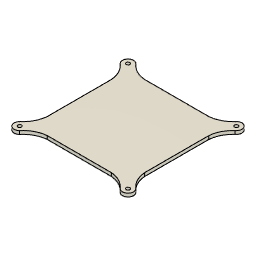
Rockin-Base (Autodesk Fusion 360 design; units mm, degrees)
Autodesk Fusion 360 part; units mm, degrees
sketch "RockinBase" plane through (-30.9845, 0, -2.9179) normal (0, 1, 0) x (-1, 0, 0)
  line L0 (109, -95) -> (109, 95)
  arc A0 (109, 95) -> (106, 98) centre (106, 95) ccw
  line L1 (106, 98) -> (-106, 98)
  arc A1 (-106, 98) -> (-109, 95) centre (-106, 95) ccw
  line L2 (-109, 95) -> (-109, -95)
  arc A2 (-109, -95) -> (-106, -98) centre (-106, -95) ccw
  line L3 (-106, -98) -> (106, -98)
  arc A3 (106, -98) -> (109, -95) centre (106, -95) ccw
  circle A4 centre (95.5, -84.5) radius 5
  circle A5 centre (95.5, 84.5) radius 5
  line L4 (-72.9845, 44) -> (11.0155, 44)
  line L5 (11.0155, -44) -> (-72.9845, -44)
  line L6 (13.0155, 42) -> (13.0155, -42)
  line L7 (-74.9845, -42) -> (-74.9845, 42)
  circle A6 centre (-79.9845, 49) radius 2.05
  circle A7 centre (-79.9845, -49) radius 2.05
  circle A8 centre (18.0155, -49) radius 2.05
  circle A9 centre (18.0155, 49) radius 2.05
  arc A10 (13.0155, 42) -> (11.0155, 44) centre (11.0155, 42) ccw
  arc A11 (11.0155, -44) -> (13.0155, -42) centre (11.0155, -42) ccw
  arc A12 (-72.9845, 44) -> (-74.9845, 42) centre (-72.9845, 42) ccw
  arc A13 (-74.9845, -42) -> (-72.9845, -44) centre (-72.9845, -42) ccw
  circle A14 centre (18.0155, -49) radius 5.05
  circle A15 centre (-79.9845, -49) radius 5.05
  circle A16 centre (-79.9845, 49) radius 5.05
  circle A17 centre (18.0155, 49) radius 5.05
  line L8 (25, -49) -> (10, -49) construction
  line L9 (18.0155, -54.05) -> (18.0155, -42) construction
  line L10 (21.6242, -45.4673) -> (14.4828, -52.6087) construction
  line L11 (21.5674, -52.5898) -> (14.4257, -45.4481) construction
  arc A18 (13.0155, -29) -> (21.6242, -45.4673) centre (36.614, -27.1472) ccw
  line L12 (13.0155, -29) -> (21.6242, -29) construction
  line L13 (21.6242, -29) -> (21.6242, -45.4673) construction
  line L14 (-1.9845, -44) -> (-1.9845, -52.6087) construction
  line L15 (-1.9845, -52.6087) -> (14.4828, -52.6087) construction
  line L16 (21.9548, -39) -> (13.0155, -39) construction
  line L17 (8.0155, -44) -> (8.0155, -52.6087) construction
  line L18 (16.1242, -39) -> (16.1242, -29) construction
  line L19 (8.0094, -47.1087) -> (-1.9845, -47.1087) construction
  arc A19 (14.4828, -52.6087) -> (-1.9845, -44) centre (-3.855, -67.6323) ccw
  arc A20 (21.6242, 45.4673) -> (13.0155, 29) centre (36.614, 27.1472) ccw
  arc A21 (-1.9845, 44) -> (14.4828, 52.6087) centre (-3.855, 67.6323) ccw
  circle A22 centre (-95.5, -84.5) radius 5
  circle A23 centre (-95.5, 84.5) radius 5
  circle A24 centre (18.0155, 49) radius 2.05
  circle A25 centre (-79.9845, 49) radius 2.05
  circle A26 centre (18.0155, -49) radius 2.05
  circle A27 centre (-79.9845, -49) radius 2.05
  line L20 (-72.9845, 44) -> (11.0155, 44)
  arc A28 (13.0155, 42) -> (11.0155, 44) centre (11.0155, 42) ccw
  line L21 (13.0155, 42) -> (13.0155, -42)
  arc A29 (11.0155, -44) -> (13.0155, -42) centre (11.0155, -42) ccw
  line L22 (11.0155, -44) -> (-72.9845, -44)
  arc A30 (-74.9845, -42) -> (-72.9845, -44) centre (-72.9845, -42) ccw
  line L23 (-74.9845, -42) -> (-74.9845, 42)
  arc A31 (-72.9845, 44) -> (-74.9845, 42) centre (-72.9845, 42) ccw
  line L24 (49.9363, -38.9018) -> (49.9363, -43.5825)
  line L25 (49.9363, -43.5825) -> (31.9363, -43.5825)
  line L26 (31.9363, -43.5825) -> (31.9363, -40.2693)
  spline S0 degree 3 poles (31.9363, -40.2693) (31.9322, -39.3416) (31.9257, -37.84) (32.1184, -36.3519) (32.192, -35.7832) knots 0 0 0 0 0.277884 0.449757 0.449757 0.449757 0.449757
  spline S1 degree 3 poles (32.192, -35.7832) (32.3135, -35.4081) (32.5613, -34.6434) (33.1821, -34.1316) (33.4984, -33.8709) knots 0 0 0 0 0.115749 0.235933 0.235933 0.235933 0.235933
  spline S2 degree 3 poles (33.4984, -33.8709) (33.9456, -33.6565) (34.9997, -33.1511) (36.1742, -33.1387) (36.8504, -33.1316) knots 0 0 0 0 0.14718 0.346909 0.346909 0.346909 0.346909
  spline S3 degree 3 poles (36.8504, -33.1316) (37.4464, -33.1268) (38.4271, -33.1191) (39.323, -33.5034) (39.6744, -33.6541) knots 0 0 0 0 0.176149 0.289849 0.289849 0.289849 0.289849
  spline S4 degree 3 poles (39.6744, -33.6541) (39.8929, -33.9007) (40.4082, -34.4822) (40.4928, -35.2619) (40.5416, -35.7109) knots 0 0 0 0 0.096727 0.228082 0.228082 0.228082 0.228082
  spline S5 degree 3 poles (40.5416, -35.7109) (40.6442, -35.307) (40.82, -34.615) (41.275, -34.07) (41.4644, -33.8431) knots 0 0 0 0 0.122975 0.210643 0.210643 0.210643 0.210643
  spline S6 degree 3 poles (41.4644, -33.8431) (41.6426, -33.7017) (41.9651, -33.4458) (42.3527, -33.3094) (42.5262, -33.2483) knots 0 0 0 0 0.067663 0.122452 0.122452 0.122452 0.122452
  spline S7 degree 3 poles (42.5262, -33.2483) (42.8284, -33.215) (43.7127, -33.1175) (44.603, -33.126) (45.1889, -33.1316) knots 0 0 0 0 0.091172 0.266721 0.266721 0.266721 0.266721
  line L27 (45.1889, -33.1316) -> (49.9363, -33.1316)
  line L28 (49.9363, -33.1316) -> (49.9363, -37.4787)
  line L29 (49.9363, -37.4787) -> (43.9548, -37.4787)
  spline S8 degree 3 poles (43.9548, -37.4787) (43.5604, -37.4703) (42.9494, -37.4573) (42.3701, -37.6414) (42.1648, -37.7066) knots 0 0 0 0 0.117155 0.181452 0.181452 0.181452 0.181452
  spline S9 degree 3 poles (42.1648, -37.7066) (42.0656, -37.8397) (41.806, -38.1877) (41.8147, -38.6291) (41.8202, -38.9018) knots 0 0 0 0 0.048702 0.127417 0.127417 0.127417 0.127417
  line L30 (41.8202, -38.9018) -> (49.9363, -38.9018)
  spline S10 degree 3 poles (35.6608, -11.9518) (35.9149, -11.5755) (36.3988, -10.8588) (37.1724, -10.4767) (37.5397, -10.2952) knots 0 0 0 0 0.133571 0.254362 0.254362 0.254362 0.254362
  spline S11 degree 3 poles (37.5397, -10.2952) (37.9942, -10.1758) (39.0458, -9.8995) (40.1346, -9.8895) (40.7528, -9.8839) knots 0 0 0 0 0.140459 0.325027 0.325027 0.325027 0.325027
  line L31 (40.7528, -9.8839) -> (40.7528, -14.1198)
  line L32 (40.7528, -14.1198) -> (39.0518, -14.1198)
  spline S12 degree 3 poles (39.0518, -14.1198) (38.8011, -14.1181) (38.3918, -14.1152) (37.998, -14.2227) (37.8455, -14.2644) knots 0 0 0 0 0.074717 0.121977 0.121977 0.121977 0.121977
  spline S13 degree 3 poles (37.8455, -14.2644) (37.7531, -14.3249) (37.5615, -14.4504) (37.5398, -14.6795) (37.5286, -14.798) knots 0 0 0 0 0.03143 0.06517 0.06517 0.06517 0.06517
  spline S14 degree 3 poles (37.5286, -14.798) (37.5364, -14.9151) (37.5509, -15.1331) (37.7256, -15.2612) (37.8066, -15.3206) knots 0 0 0 0 0.033254 0.06196 0.06196 0.06196 0.06196
  spline S15 degree 3 poles (37.8066, -15.3206) (37.956, -15.3589) (38.3632, -15.4632) (38.7849, -15.4576) (39.0518, -15.454) knots 0 0 0 0 0.046126 0.12569 0.12569 0.12569 0.12569
  line L33 (39.0518, -15.454) -> (46.0116, -15.454)
  spline S16 degree 3 poles (46.0116, -15.454) (46.2446, -15.4518) (46.6509, -15.4479) (47.0327, -15.3119) (47.1957, -15.2539) knots 0 0 0 0 0.069251 0.12082 0.12082 0.12082 0.12082
  spline S17 degree 3 poles (47.1957, -15.2539) (47.3108, -15.1821) (47.532, -15.0441) (47.5714, -14.7877) (47.5904, -14.6646) knots 0 0 0 0 0.038577 0.07416 0.07416 0.07416 0.07416
  spline S18 degree 3 poles (47.5904, -14.6646) (47.574, -14.5252) (47.5414, -14.2493) (47.299, -14.1143) (47.179, -14.0476) knots 0 0 0 0 0.039578 0.078352 0.078352 0.078352 0.078352
  spline S19 degree 3 poles (47.179, -14.0476) (46.9815, -14.0011) (46.4708, -13.881) (45.945, -13.8843) (45.6225, -13.8864) knots 0 0 0 0 0.060698 0.156952 0.156952 0.156952 0.156952
  line L34 (45.6225, -13.8864) -> (43.8659, -13.8864)
  line L35 (43.8659, -13.8864) -> (43.8659, -9.8839)
  spline S20 degree 3 poles (43.8659, -9.8839) (44.3819, -9.8878) (45.2677, -9.8945) (46.1495, -9.9772) (46.5175, -10.0117) knots 0 0 0 0 0.154724 0.265578 0.265578 0.265578 0.265578
  spline S21 degree 3 poles (46.5175, -10.0117) (46.8221, -10.0776) (47.4698, -10.2177) (48.032, -10.57) (48.3297, -10.7566) knots 0 0 0 0 0.092782 0.197263 0.197263 0.197263 0.197263
  spline S22 degree 3 poles (48.3297, -10.7566) (48.6201, -10.9818) (49.2003, -11.4318) (49.5539, -12.0752) (49.7306, -12.3965) knots 0 0 0 0 0.108972 0.217725 0.217725 0.217725 0.217725
  spline S23 degree 3 poles (49.7306, -12.3965) (49.8682, -12.7698) (50.1655, -13.5761) (50.19, -14.4361) (50.2031, -14.8981) knots 0 0 0 0 0.118546 0.256084 0.256084 0.256084 0.256084
  spline S24 degree 3 poles (50.2031, -14.8981) (50.1888, -15.4752) (50.1629, -16.5234) (49.7419, -17.4808) (49.5527, -17.9111) knots 0 0 0 0 0.171157 0.310864 0.310864 0.310864 0.310864
  spline S25 degree 3 poles (49.5527, -17.9111) (49.3153, -18.2541) (48.8433, -18.9362) (48.0992, -19.3023) (47.7294, -19.4843) knots 0 0 0 0 0.122923 0.244404 0.244404 0.244404 0.244404
  spline S26 degree 3 poles (47.7294, -19.4843) (47.2592, -19.6182) (46.1727, -19.9278) (45.0413, -19.9392) (44.3995, -19.9456) knots 0 0 0 0 0.146052 0.33749 0.33749 0.33749 0.33749
  line L36 (44.3995, -19.9456) -> (40.2081, -19.9456)
  spline S27 degree 3 poles (40.2081, -19.9456) (39.6546, -19.9419) (38.692, -19.9352) (37.7664, -19.6773) (37.373, -19.5676) knots 0 0 0 0 0.165095 0.287118 0.287118 0.287118 0.287118
  spline S28 degree 3 poles (37.373, -19.5676) (37.0535, -19.3898) (36.3506, -18.9987) (35.9079, -18.3237) (35.6664, -17.9555) knots 0 0 0 0 0.108122 0.237874 0.237874 0.237874 0.237874
  spline S29 degree 3 poles (35.6664, -17.9555) (35.4476, -17.5077) (34.9856, -16.5617) (34.9399, -15.5084) (34.9159, -14.9537) knots 0 0 0 0 0.147881 0.312389 0.312389 0.312389 0.312389
  spline S30 degree 3 poles (34.9159, -14.9537) (34.9402, -14.4011) (34.9865, -13.3489) (35.4437, -12.4016) (35.6608, -11.9518) knots 0 0 0 0 0.163939 0.312177 0.312177 0.312177 0.312177
  line L37 (35.5385, 37.6788) -> (33.2148, 37.6788)
  line L38 (33.2148, 37.6788) -> (33.2148, 42.1816)
  line L39 (33.2148, 42.1816) -> (35.5385, 42.1816)
  line L40 (35.5385, 42.1816) -> (35.5385, 43.3935)
  line L41 (35.5385, 43.3935) -> (37.8733, 43.3935)
  line L42 (37.8733, 43.3935) -> (37.8733, 42.1816)
  line L43 (37.8733, 42.1816) -> (45.767, 42.1816)
  spline S31 degree 3 poles (45.767, 42.1816) (46.1483, 42.169) (46.6983, 42.1509) (47.2278, 42.2893) (47.3903, 42.3317) knots 0 0 0 0 0.113465 0.163663 0.163663 0.163663 0.163663
  spline S32 degree 3 poles (47.3903, 42.3317) (47.4376, 42.4599) (47.5853, 42.8601) (47.5685, 43.2902) (47.557, 43.5825) knots 0 0 0 0 0.040741 0.127145 0.127145 0.127145 0.127145
  line L44 (47.557, 43.5825) -> (49.9363, 43.5825)
  line L45 (49.9363, 43.5825) -> (49.9363, 41.7702)
  spline S33 degree 3 poles (49.9363, 41.7702) (49.9367, 41.3313) (49.9375, 40.5983) (49.8454, 39.8715) (49.8084, 39.58) knots 0 0 0 0 0.131509 0.219587 0.219587 0.219587 0.219587
  spline S34 degree 3 poles (49.8084, 39.58) (49.7515, 39.3674) (49.6372, 38.9402) (49.359, 38.5964) (49.2192, 38.4237) knots 0 0 0 0 0.06522 0.131072 0.131072 0.131072 0.131072
  spline S35 degree 3 poles (49.2192, 38.4237) (49.063, 38.2734) (48.76, 37.9817) (48.3579, 37.8601) (48.163, 37.8011) knots 0 0 0 0 0.063989 0.124175 0.124175 0.124175 0.124175
  spline S36 degree 3 poles (48.163, 37.8011) (47.8311, 37.7661) (46.9021, 37.6681) (45.9675, 37.6746) (45.3668, 37.6788) knots 0 0 0 0 0.100066 0.280064 0.280064 0.280064 0.280064
  line L46 (45.3668, 37.6788) -> (37.8733, 37.6788)
  line L47 (37.8733, 37.6788) -> (37.8733, 36.7116)
  line L48 (37.8733, 36.7116) -> (35.5385, 36.7116)
  line L49 (35.5385, 36.7116) -> (35.5385, 37.6788)
  line L50 (49.9363, 13.9753) -> (31.9363, 13.9753)
  line L51 (31.9363, 13.9753) -> (31.9363, 18.467)
  line L52 (31.9363, 18.467) -> (36.1972, 18.467)
  spline S37 degree 3 poles (36.1972, 18.467) (35.9973, 18.6537) (35.6098, 19.0158) (35.3562, 19.4813) (35.2335, 19.7066) knots 0 0 0 0 0.081471 0.157931 0.157931 0.157931 0.157931
  spline S38 degree 3 poles (35.2335, 19.7066) (35.1408, 19.9414) (34.9527, 20.4184) (34.9283, 20.9307) (34.9159, 21.1909) knots 0 0 0 0 0.075167 0.152706 0.152706 0.152706 0.152706
  spline S39 degree 3 poles (34.9159, 21.1909) (34.9249, 21.4809) (34.942, 22.0293) (35.1207, 22.5476) (35.205, 22.7918) knots 0 0 0 0 0.086467 0.163515 0.163515 0.163515 0.163515
  spline S40 degree 3 poles (35.205, 22.7918) (35.3072, 23.0018) (35.5037, 23.4053) (35.8503, 23.6895) (36.0166, 23.8258) knots 0 0 0 0 0.069125 0.132834 0.132834 0.132834 0.132834
  spline S41 degree 3 poles (36.0166, 23.8258) (36.1844, 23.9317) (36.5017, 24.132) (36.8672, 24.2148) (37.0394, 24.2539) knots 0 0 0 0 0.059029 0.111602 0.111602 0.111602 0.111602
  spline S42 degree 3 poles (37.0394, 24.2539) (37.3006, 24.2746) (38.0108, 24.331) (38.7235, 24.328) (39.1741, 24.3261) knots 0 0 0 0 0.078569 0.213664 0.213664 0.213664 0.213664
  line L53 (39.1741, 24.3261) -> (45.8226, 24.3261)
  spline S43 degree 3 poles (45.8226, 24.3261) (46.2964, 24.3248) (47.1094, 24.3226) (47.9076, 24.1721) (48.2408, 24.1093) knots 0 0 0 0 0.141719 0.24323 0.24323 0.24323 0.24323
  spline S44 degree 3 poles (48.2408, 24.1093) (48.5013, 24.0066) (49.0498, 23.7903) (49.4233, 23.3324) (49.6194, 23.092) knots 0 0 0 0 0.082602 0.173904 0.173904 0.173904 0.173904
  spline S45 degree 3 poles (49.6194, 23.092) (49.7896, 22.8078) (50.14, 22.2226) (50.1817, 21.5412) (50.2031, 21.1909) knots 0 0 0 0 0.097889 0.201485 0.201485 0.201485 0.201485
  spline S46 degree 3 poles (50.2031, 21.1909) (50.1892, 20.933) (50.1615, 20.4214) (49.9585, 19.9511) (49.8578, 19.7177) knots 0 0 0 0 0.076784 0.152376 0.152376 0.152376 0.152376
  spline S47 degree 3 poles (49.8578, 19.7177) (49.724, 19.4912) (49.4454, 19.0195) (49.035, 18.6559) (48.8217, 18.467) knots 0 0 0 0 0.078411 0.163305 0.163305 0.163305 0.163305
  line L54 (48.8217, 18.467) -> (49.9363, 18.1779)
  line L55 (49.9363, 18.1779) -> (49.9363, 13.9753)
  spline S48 degree 3 poles (36.5391, 34.9438) (36.7763, 35.1231) (37.2322, 35.4677) (37.7706, 35.6584) (38.0289, 35.7498) knots 0 0 0 0 0.088578 0.170285 0.170285 0.170285 0.170285
  spline S49 degree 3 poles (38.0289, 35.7498) (38.3505, 35.8127) (39.1206, 35.9631) (39.9061, 35.9653) (40.3637, 35.9666) knots 0 0 0 0 0.098084 0.234942 0.234942 0.234942 0.234942
  line L56 (40.3637, 35.9666) -> (43.977, 35.9666)
  spline S50 degree 3 poles (43.977, 35.9666) (44.5532, 35.9662) (45.5311, 35.9654) (46.4982, 35.8244) (46.8955, 35.7665) knots 0 0 0 0 0.17254 0.292859 0.292859 0.292859 0.292859
  spline S51 degree 3 poles (46.8955, 35.7665) (47.2029, 35.6784) (47.8324, 35.4978) (48.3599, 35.1093) (48.6299, 34.9104) knots 0 0 0 0 0.095113 0.194798 0.194798 0.194798 0.194798
  spline S52 degree 3 poles (48.6299, 34.9104) (48.8819, 34.6739) (49.3932, 34.1938) (49.6761, 33.5517) (49.8195, 33.2261) knots 0 0 0 0 0.102553 0.208104 0.208104 0.208104 0.208104
  spline S53 degree 3 poles (49.8195, 33.2261) (49.9313, 32.8604) (50.1667, 32.0909) (50.1906, 31.286) (50.2031, 30.8635) knots 0 0 0 0 0.114169 0.240306 0.240306 0.240306 0.240306
  spline S54 degree 3 poles (50.2031, 30.8635) (50.1944, 30.4023) (50.1782, 29.5484) (49.9706, 28.7205) (49.8751, 28.3397) knots 0 0 0 0 0.137828 0.255228 0.255228 0.255228 0.255228
  spline S55 degree 3 poles (49.8751, 28.3397) (49.7588, 28.0205) (49.5386, 27.4162) (49.0949, 26.9521) (48.8856, 26.7332) knots 0 0 0 0 0.100653 0.190512 0.190512 0.190512 0.190512
  spline S56 degree 3 poles (48.8856, 26.7332) (48.6495, 26.5549) (48.1642, 26.1886) (47.5831, 26.0085) (47.2846, 25.916) knots 0 0 0 0 0.088036 0.180963 0.180963 0.180963 0.180963
  spline S57 degree 3 poles (47.2846, 25.916) (46.8941, 25.8451) (45.9631, 25.6761) (45.0161, 25.6731) (44.4662, 25.6714) knots 0 0 0 0 0.118858 0.283378 0.283378 0.283378 0.283378
  line L57 (44.4662, 25.6714) -> (40.6861, 25.6714)
  spline S58 degree 3 poles (40.6861, 25.6714) (40.0711, 25.6784) (38.9797, 25.691) (37.9308, 25.9869) (37.473, 26.1161) knots 0 0 0 0 0.183506 0.325616 0.325616 0.325616 0.325616
  spline S59 degree 3 poles (37.473, 26.1161) (37.104, 26.2984) (36.348, 26.6718) (35.864, 27.3632) (35.6163, 27.7171) knots 0 0 0 0 0.12141 0.248708 0.248708 0.248708 0.248708
  spline S60 degree 3 poles (35.6163, 27.7171) (35.4123, 28.1491) (34.9712, 29.0834) (34.9352, 30.1182) (34.9159, 30.6745) knots 0 0 0 0 0.141834 0.306758 0.306758 0.306758 0.306758
  spline S61 degree 3 poles (34.9159, 30.6745) (34.9293, 31.1472) (34.9544, 32.035) (35.235, 32.8769) (35.3662, 33.2705) knots 0 0 0 0 0.140953 0.26475 0.26475 0.26475 0.26475
  spline S62 degree 3 poles (35.3662, 33.2705) (35.5196, 33.6045) (35.809, 34.2345) (36.3057, 34.717) (36.5391, 34.9438) knots 0 0 0 0 0.109129 0.205914 0.205914 0.205914 0.205914
  spline S63 degree 3 poles (36.5391, 11.4737) (36.7763, 11.653) (37.2322, 11.9976) (37.7706, 12.1883) (38.0289, 12.2798) knots 0 0 0 0 0.088577 0.170285 0.170285 0.170285 0.170285
  spline S64 degree 3 poles (38.0289, 12.2798) (38.3505, 12.3426) (39.1206, 12.4931) (39.9061, 12.4953) (40.3637, 12.4966) knots 0 0 0 0 0.098084 0.234942 0.234942 0.234942 0.234942
  line L58 (40.3637, 12.4966) -> (43.977, 12.4966)
  spline S65 degree 3 poles (43.977, 12.4966) (44.5532, 12.4961) (45.5311, 12.4954) (46.4982, 12.3544) (46.8955, 12.2965) knots 0 0 0 0 0.17254 0.292859 0.292859 0.292859 0.292859
  spline S66 degree 3 poles (46.8955, 12.2965) (47.2029, 12.2083) (47.8324, 12.0277) (48.3599, 11.6392) (48.6299, 11.4404) knots 0 0 0 0 0.095113 0.194798 0.194798 0.194798 0.194798
  spline S67 degree 3 poles (48.6299, 11.4404) (48.8819, 11.2038) (49.3932, 10.7237) (49.6761, 10.0817) (49.8195, 9.756) knots 0 0 0 0 0.102553 0.208104 0.208104 0.208104 0.208104
  spline S68 degree 3 poles (49.8195, 9.756) (49.9313, 9.3904) (50.1667, 8.6208) (50.1906, 7.8159) (50.2031, 7.3935) knots 0 0 0 0 0.114169 0.240305 0.240305 0.240305 0.240305
  spline S69 degree 3 poles (50.2031, 7.3935) (50.1944, 6.9323) (50.1782, 6.0784) (49.9706, 5.2505) (49.8751, 4.8697) knots 0 0 0 0 0.137829 0.255229 0.255229 0.255229 0.255229
  spline S70 degree 3 poles (49.8751, 4.8697) (49.7588, 4.5504) (49.5386, 3.9462) (49.0949, 3.482) (48.8856, 3.2631) knots 0 0 0 0 0.100652 0.190512 0.190512 0.190512 0.190512
  spline S71 degree 3 poles (48.8856, 3.2631) (48.6495, 3.0849) (48.1642, 2.7186) (47.5831, 2.5384) (47.2846, 2.446) knots 0 0 0 0 0.088036 0.180963 0.180963 0.180963 0.180963
  spline S72 degree 3 poles (47.2846, 2.446) (46.8941, 2.3751) (45.9631, 2.2061) (45.0161, 2.2031) (44.4662, 2.2014) knots 0 0 0 0 0.118858 0.283378 0.283378 0.283378 0.283378
  line L59 (44.4662, 2.2014) -> (40.6861, 2.2014)
  spline S73 degree 3 poles (40.6861, 2.2014) (40.0711, 2.2084) (38.9797, 2.2209) (37.9308, 2.5169) (37.473, 2.6461) knots 0 0 0 0 0.183506 0.325616 0.325616 0.325616 0.325616
  spline S74 degree 3 poles (37.473, 2.6461) (37.104, 2.8283) (36.348, 3.2017) (35.864, 3.8932) (35.6163, 4.2471) knots 0 0 0 0 0.121411 0.248708 0.248708 0.248708 0.248708
  spline S75 degree 3 poles (35.6163, 4.2471) (35.4123, 4.6791) (34.9712, 5.6134) (34.9352, 6.6481) (34.9159, 7.2044) knots 0 0 0 0 0.141835 0.306758 0.306758 0.306758 0.306758
  spline S76 degree 3 poles (34.9159, 7.2044) (34.9293, 7.6771) (34.9544, 8.565) (35.235, 9.4068) (35.3662, 9.8005) knots 0 0 0 0 0.140953 0.26475 0.26475 0.26475 0.26475
  spline S77 degree 3 poles (35.3662, 9.8005) (35.5196, 10.1344) (35.809, 10.7645) (36.3057, 11.247) (36.5391, 11.4737) knots 0 0 0 0 0.109129 0.205915 0.205915 0.205915 0.205915
  line L60 (39.4925, -4.0525) -> (35.1827, -2.6516)
  line L61 (35.1827, -2.6516) -> (35.1827, 1.1229)
  line L62 (35.1827, 1.1229) -> (41.0586, -0.7004)
  line L63 (41.0586, -0.7004) -> (49.9363, 1.6677)
  line L64 (49.9363, 1.6677) -> (49.9363, -2.6516)
  line L65 (49.9363, -2.6516) -> (43.5061, -4.0525)
  line L66 (43.5061, -4.0525) -> (49.9363, -4.0581)
  line L67 (49.9363, -4.0581) -> (49.9363, -8.5497)
  line L68 (49.9363, -8.5497) -> (31.9363, -8.5497)
  line L69 (31.9363, -8.5497) -> (31.9363, -4.0581)
  line L70 (31.9363, -4.0581) -> (39.4925, -4.0525)
  spline S78 degree 3 poles (36.5391, -22.3138) (36.7763, -22.1345) (37.2322, -21.7899) (37.7706, -21.5992) (38.0289, -21.5077) knots 0 0 0 0 0.088577 0.170285 0.170285 0.170285 0.170285
  spline S79 degree 3 poles (38.0289, -21.5077) (38.3505, -21.4449) (39.1206, -21.2945) (39.9061, -21.2922) (40.3637, -21.2909) knots 0 0 0 0 0.098084 0.234942 0.234942 0.234942 0.234942
  line L71 (40.3637, -21.2909) -> (43.977, -21.2909)
  spline S80 degree 3 poles (43.977, -21.2909) (44.5532, -21.2914) (45.5311, -21.2921) (46.4982, -21.4331) (46.8955, -21.491) knots 0 0 0 0 0.17254 0.292859 0.292859 0.292859 0.292859
  spline S81 degree 3 poles (46.8955, -21.491) (47.2029, -21.5792) (47.8324, -21.7598) (48.3599, -22.1483) (48.6299, -22.3471) knots 0 0 0 0 0.095113 0.194798 0.194798 0.194798 0.194798
  spline S82 degree 3 poles (48.6299, -22.3471) (48.8819, -22.5837) (49.3932, -23.0638) (49.6761, -23.7058) (49.8195, -24.0315) knots 0 0 0 0 0.102553 0.208104 0.208104 0.208104 0.208104
  spline S83 degree 3 poles (49.8195, -24.0315) (49.9313, -24.3971) (50.1667, -25.1667) (50.1906, -25.9716) (50.2031, -26.3941) knots 0 0 0 0 0.114169 0.240306 0.240306 0.240306 0.240306
  spline S84 degree 3 poles (50.2031, -26.3941) (50.1944, -26.8552) (50.1782, -27.7092) (49.9706, -28.537) (49.8751, -28.9179) knots 0 0 0 0 0.137829 0.255228 0.255228 0.255228 0.255228
  spline S85 degree 3 poles (49.8751, -28.9179) (49.7588, -29.2371) (49.5386, -29.8414) (49.0949, -30.3055) (48.8856, -30.5244) knots 0 0 0 0 0.100652 0.190512 0.190512 0.190512 0.190512
  spline S86 degree 3 poles (48.8856, -30.5244) (48.6495, -30.7026) (48.1642, -31.069) (47.5831, -31.2491) (47.2846, -31.3416) knots 0 0 0 0 0.088036 0.180963 0.180963 0.180963 0.180963
  spline S87 degree 3 poles (47.2846, -31.3416) (46.8941, -31.4125) (45.9631, -31.5815) (45.0161, -31.5844) (44.4662, -31.5862) knots 0 0 0 0 0.118858 0.283378 0.283378 0.283378 0.283378
  line L72 (44.4662, -31.5862) -> (40.6861, -31.5862)
  spline S88 degree 3 poles (40.6861, -31.5862) (40.0711, -31.5791) (38.9797, -31.5666) (37.9308, -31.2706) (37.473, -31.1414) knots 0 0 0 0 0.183506 0.325616 0.325616 0.325616 0.325616
  spline S89 degree 3 poles (37.473, -31.1414) (37.104, -30.9592) (36.348, -30.5858) (35.864, -29.8944) (35.6163, -29.5405) knots 0 0 0 0 0.12141 0.248708 0.248708 0.248708 0.248708
  spline S90 degree 3 poles (35.6163, -29.5405) (35.4123, -29.1085) (34.9712, -28.1741) (34.9352, -27.1394) (34.9159, -26.5831) knots 0 0 0 0 0.141835 0.306757 0.306757 0.306757 0.306757
  spline S91 degree 3 poles (34.9159, -26.5831) (34.9293, -26.1104) (34.9544, -25.2225) (35.235, -24.3807) (35.3662, -23.987) knots 0 0 0 0 0.140954 0.26475 0.26475 0.26475 0.26475
  spline S92 degree 3 poles (35.3662, -23.987) (35.5196, -23.6531) (35.809, -23.023) (36.3057, -22.5406) (36.5391, -22.3138) knots 0 0 0 0 0.109129 0.205915 0.205915 0.205915 0.205915
  line L73 (13.0155, 0) -> (-74.9845, 0) construction
  line L74 (-30.9845, -44) -> (-30.9845, 44) construction
  arc A32 (-83.5932, -45.4673) -> (-74.9845, -29) centre (-98.583, -27.1472) ccw
  arc A33 (-59.9845, -44) -> (-76.4518, -52.6087) centre (-58.114, -67.6323) ccw
  arc A34 (-74.9845, 29) -> (-83.5932, 45.4673) centre (-98.583, 27.1472) ccw
  arc A35 (-76.4518, 52.6087) -> (-59.9845, 44) centre (-58.114, 67.6323) ccw
  circle A36 centre (18.0155, -49) radius 1.55
  circle A37 centre (-79.9845, -49) radius 1.55
  circle A38 centre (-79.9845, 49) radius 1.55
  circle A39 centre (18.0155, 49) radius 1.55
  circle A40 centre (95.5, -84.5) radius 1.55
  dimension "d192" = 3
  dimension "d193" = 45
  dimension "d194" = 45
  dimension "d195" = 20
  dimension "d197" = 20
  dimension "d198" = 10
  dimension "d200" = 10
  dimension "d201" = 5.5
  dimension "d202" = 5.5
  constraint concentric A7 A15
  constraint concentric A6 A16
  constraint concentric A9 A17
  constraint equal A14 A17
  constraint equal A15 A16
  constraint equal A14 A15
  constraint horizontal L8
  constraint coincident A14 L9.start
  constraint perpendicular L8 L9
  constraint coincident A14 L10.start
  constraint coincident A14 L10.end
  constraint coincident A14 L11.start
  constraint coincident A14 L11.end
  constraint coincident L6 A18.start
  constraint perpendicular L6 L12
  constraint coincident L5 L14.start
  constraint perpendicular L5 L14
  constraint coincident L6 L16.end
  constraint perpendicular L6 L16
  constraint coincident L15 L17.end
  constraint perpendicular L15 L17
  constraint parallel L14 L17
  constraint coincident A18 L18.start
  constraint coincident L16 L18.start
  constraint coincident L12 L18.end
  constraint perpendicular L12 L18
  constraint parallel L13 L18
  constraint coincident L19.start A19
  constraint midpoint L21 L73.start
  constraint midpoint L23 L73.end
  constraint midpoint L5 L74.start
  constraint midpoint L20 L74.end
  constraint symmetric L10.start L74 A32.start
  constraint symmetric L10.end L74 A33.end
  constraint symmetric A18.start L74 A32.end
  constraint symmetric A18 L74 A32
  constraint symmetric L14.start L74 A33.start
  constraint symmetric A19 L74 A33
  constraint symmetric A20.end L74 A34.start
  constraint symmetric A20.start L74 A34.end
  constraint symmetric A20 L74 A34
  constraint symmetric A21.end L74 A35.start
  constraint symmetric A21.start L74 A35.end
  constraint symmetric A21 L74 A35
  constraint concentric A26 A36
  constraint concentric A15 A37
  constraint concentric A6 A38
  constraint concentric A24 A39
  constraint equal A36 A39
  constraint equal A38 A39
  constraint equal A37 A38
  constraint equal A36 A40
  measures "d192" distance of A8 A14
  measures "d193" angle of L9 L10
  measures "d194" angle of L8 L11
  measures "d195" distance of A8.centre L12
  measures "d197" distance of A8.centre L14
  measures "d198" distance of L12 L16
  measures "d200" distance of L14 L17
  measures "d201" distance of L13 L18
  measures "d202" distance of L15 L19
extrude "Extrude2" add sketch "RockinBase" along normal blind 3 contours L4 L7 A12 A16 L20 L23 A31 A34 A35 | L4 L5 L6 L7 A10 A11 A12 A13 L20 A28 L21 A29 L22 A30 L23 A31 | L4 L6 A10 A17 A20 A21 L20 A28 L21 | A16 A35 | A16 A34 A35 | A17 A20 A21 | L5 L7 A13 A15 L22 A30 L23 A32 A33 | A16 A34 | A15 A32 | A15 A32 A33 | L5 L6 A11 A14 A18 A19 L21 A29 L22 | A15 A33 | A14 A18 A19 | A6 A25 | A7 A27 | A8 A26 | A9 A24
sketch "EnlargedHoles" plane through (0, 3, 0) normal (0, 1, 0) x (-1, 0, 0)
  circle A0 centre (-49, -51.9179) radius 1.55
  circle A1 centre (49, -51.9179) radius 1.55
  circle A2 centre (49, 46.0821) radius 1.55
  circle A3 centre (-49, 46.0821) radius 1.55
  arc A4 (-51.9103, -47.7909) -> (-44.8759, -54.8324) centre (-49, -51.9179) ccw
  arc A5 (-29, -46.9179) -> (-44.8759, -54.8324) centre (-27.1295, -70.5502) ccw
  line L0 (-29, -46.9179) -> (29, -46.9179)
  arc A6 (45.4673, -55.5266) -> (29, -46.9179) centre (27.1295, -70.5502) ccw
  arc A7 (45.4673, -55.5266) -> (52.6087, -48.3853) centre (49, -51.9179) ccw
  arc A8 (44, -31.9179) -> (52.6087, -48.3853) centre (67.5985, -30.0651) ccw
  line L1 (44, -31.9179) -> (44, 26.0821)
  arc A9 (52.6087, 42.5494) -> (44, 26.0821) centre (67.5985, 24.2292) ccw
  arc A10 (52.6087, 42.5494) -> (45.4673, 49.6907) centre (49, 46.0821) ccw
  arc A11 (29, 41.0821) -> (45.4673, 49.6907) centre (27.1295, 64.7143) ccw
  line L2 (29, 41.0821) -> (-29, 41.0821)
  arc A12 (-44.8759, 48.9965) -> (-29, 41.0821) centre (-27.1295, 64.7143) ccw
  arc A13 (-44.8759, 48.9965) -> (-51.9103, 41.955) centre (-49, 46.0821) ccw
  arc A14 (-44, 26.0821) -> (-51.9103, 41.955) centre (-67.5985, 24.2292) ccw
  line L3 (-44, 26.0821) -> (-44, -31.9179)
  arc A15 (-51.9103, -47.7909) -> (-44, -31.9179) centre (-67.5985, -30.0651) ccw
  circle A16 centre (49, -51.9179) radius 1.65
  circle A17 centre (-49, -51.9179) radius 1.65
  circle A18 centre (-49, 46.0821) radius 1.65
  circle A19 centre (49, 46.0821) radius 1.65
  dimension "d1" = 3.3
  constraint concentric A1 A16
  constraint concentric A0 A17
  constraint concentric A3 A18
  constraint concentric A2 A19
  constraint equal A17 A19
  constraint equal A16 A17
  constraint equal A18 A19
  measures "d1" diameter of A16
extrude "Extrude3" cut sketch "EnlargedHoles" against normal up to surface (3 mm away) contours A16 | A17 | A18 | A19
